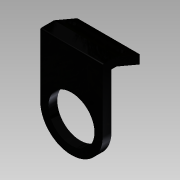
# Autodesk Inventor part: Dudukan Proximity V3
Saved by Autodesk Inventor 2015 SP1 (Build 190203100, 203)
## iProperties
Created: 2015-01-10
Part Number: Dudukan Proximity V3
Material: Generic
Document SubType Name: Modeling
Designer: Rafi Kurnia Putra
Density: 1 g/cm^3
Appearance: Smooth - Purple
Mass: 1.16017 g
Surface Area: 15.749 cm^2
Volume: 1.16017 cm^3
Author: Rafi Kurnia Putra
Autodesk Inventor part; units mm, degrees
ref_plane "YZ Plane" through (0, 0, 0) normal (1, 0, 0) x (0, 1, 0)
ref_plane "XZ Plane" through (0, 0, 0) normal (0, 1, 0) x (-1, 0, 0)
ref_plane "XY Plane" through (0, 0, 0) normal (0, 0, 1) x (1, 0, 0)
sketch "Sketch1" plane through (0, 0, 0) normal (0, 0, 1) x (1, 0, 0)
  circle A0 centre (0, 25) radius 9.125
  line L0 (-12.375, 0) -> (12.375, 0)
  arc A1 (12.375, 25) -> (-12.375, 25) centre (0, 25) ccw
  line L1 (12.375, 0) -> (12.375, 25)
  line L2 (-12.375, 0) -> (-12.375, 25)
  point P0 (0, 0)
  dimension "d28" = 18.25
  dimension "d29" = 24.75
  dimension "d30" = 24.75
  dimension "d70" = 25
  dimension "d71" = 25
  constraints: 6 end point, 2 centre point, 2 horizontal, 2 point on circle, 2 tangent, 1 coincident, 1 midpoint
  measures "d28" diameter of A0
  measures "d29" diameter of A1
  measures "d30" distance of L0.start L0.end
  measures "d70" distance of L0.start L2.end
  measures "d71" distance of L0.end L1.end
extrude "Extrusion5" add sketch "Sketch1" against normal blind 3.5
fillet "Fillet1" radius 0.5 1 edges at (0, 0, 0)
sketch "Sketch3" plane through (0, 0, -3.5) normal (0, 0, -1) x (-1, 0, 0)
  line L0 (12.375, 0) -> (12.375, 25) projected
  line L1 (-12.375, 25) -> (-12.375, 0) projected
  line L2 (-12.375, 0) -> (12.375, 0) projected
  line L3 (12.375, 0) -> (-12.375, 0)
  line L4 (-12.375, 0) -> (-12.375, 3.5)
  line L5 (-12.375, 3.5) -> (12.375, 3.5)
  line L6 (12.375, 3.5) -> (12.375, 0)
  point P0 (0, 0)
  dimension "d54" = 3.5
  constraints: 8 end point, 2 parallel, 1 horizontal, 1 perpendicular, 1 point on line
  measures "d54" distance of L3.end L4.end
sketch "Sketch4" plane through (12.375, 0, -3.5) normal (1, 0, 0) x (0, 0, -1)
  line L0 (0, 0) -> (10, 0) construction
  line L1 (0, 0) -> (2, 0)
  line L2 (2, 0) -> (11.205, 3.9073)
  line L3 (2, 0) -> (12, 0) construction
  point P0 (-2, 0)
  dimension "d67" = 10
  dimension "d68" = 23
  constraints: 8 end point, 2 horizontal, 1 equal length, 1 point on line
  measures "d67" distance of L1.end L2.end
  measures "d68" angle of L3 L2
sweep "Sweep1" add profiles "Sketch3" path "Sketch4" keep normal constant yes
sketch "Sketch6" plane through (-12.375, 0, -5.5) normal (0, -0.9205049, -0.3907311) x (1, 0, 0)
  circle A0 centre (3, -5) radius 1.5
  circle A1 centre (21.75, -5) radius 1.5
  line L0 (0, 0) -> (0, -10) projected
  line L1 (24.75, 0) -> (24.75, -10) projected
  line L2 (24.75, 0) -> (0, 0) projected
  line L3 (24.75, -10) -> (0, -10) projected
  point P0 (12.375, 5.0628)
  dimension "d72" = 3
  dimension "d73" = 3
  dimension "d74" = 3
  dimension "d75" = 3
  dimension "d76" = 5
  dimension "d77" = 5
  dimension "d78" = 5
  constraints: 2 centre point
  measures "d72" diameter of A0
  measures "d73" diameter of A1
  measures "d74" distance from line of A0.centre L0
  measures "d75" distance from line of A1.centre L1
  measures "d76" distance from line of A0.centre L2
  measures "d77" distance from line of L3 A0.centre
  measures "d78" distance from line of A1.centre L2
extrude "Extrusion7" cut sketch "Sketch6" against normal up to next contours A0 | A1
equation "\"d71\" = d70"
equation "\"d75\" = d74"
equation "\"d78\" = d76"
body "Solid3"
